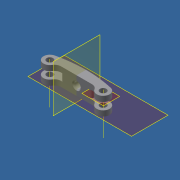
# Autodesk Inventor part: Hebel_B dual
Saved by Autodesk Inventor 2016 (Build 200138000, 138)
## iProperties
Created: 2014-12-22
Part Number: Hebel_B dual
Material: Generisch
Document SubType Name: Modeling
Designer: 4ndreas
Density: 1 g/cm^3
Appearance: Vorgabe
Mass: 1.35892 g
Surface Area: 18.535 cm^2
Volume: 1.35892 cm^3
Author: 4ndreas
Autodesk Inventor part; units mm, degrees
ref_plane "YZ Plane" through (0, 0, 0) normal (1, 0, 0) x (0, 1, 0)
ref_plane "XZ Plane" through (0, 0, 0) normal (0, 1, 0) x (-1, 0, 0)
ref_plane "XY Plane" through (0, 0, 0) normal (0, 0, 1) x (1, 0, 0)
sketch "Skizze1" plane through (0, 0, 0) normal (0, 0, 1) x (1, 0, 0)
  line L0 (0, 0) -> (25, 0) construction
  arc A0 (0, 3) -> (2.5981, -1.5) centre (0, 0) ccw
  arc A1 (22.4019, -1.5) -> (25, 3) centre (25, 0) ccw
  arc A2 (22.4019, -1.5) -> (19.8038, 0) centre (19.8038, -3) ccw
  arc A3 (5.1962, 0) -> (2.5981, -1.5) centre (5.1962, -3) ccw
  line L1 (0, 3) -> (25, 3)
  line L2 (5.1962, 0) -> (19.8038, 0)
  line L3 (12.5, 0) -> (12.5, 11.1623) construction
  line L4 (-0.6713, 2.9239) -> (12.5, 5.9481) construction
  line L5 (12.5, 5.9481) -> (25.6713, 2.9239) construction
  spline S0 degree 2 poles (-0.6713, 2.9239) (12.5, 5.9481) (25.6713, 2.9239) knots 1 1 1 2 2 2
  dimension "d0" = 25
  dimension "d1" = 3
  dimension "d2" = 3
  constraints: 10 point on circle, 8 end point, 8 tangent, 4 centre point, 2 coincident, 1 collinear, 1 equal radius, 1 horizontal, 1 midpoint, 1 parallel, 1 perpendicular, 1 point on line, 4 other
  measures "d0" distance of L0.start L0.end
  measures "d1" radius of A0
  measures "d2" distance between parallel lines of L2 L1
ref_plane "Arbeitsebene1" through (0, 3, 0) normal (0, 0, -1) x (1, 0, 0)
extrude "Extrusion1" add sketch "Skizze1" along normal blind 2.5
sketch "Skizze2" plane through (0, 0, 2.5) normal (0, 0, 1) x (1, 0, 0)
  arc A0 (-0.6713, 2.9239) -> (2.5981, -1.5) centre (0, 0) ccw projected
  arc A1 (22.4019, -1.5) -> (25.6713, 2.9239) centre (25, 0) ccw projected
  point P0 (0, 3)
  point P1 (25, 3)
hole "Bohrung1" at (0, 0, 2.5) at (25, 0, 2.5) direction (0, 0, -1) diameter 3 end through all
sketch "Skizze4" plane through (0, 0, 2.5) normal (0, 0, 1) x (1, 0, 0)
  line L0 (5.1962, 0) -> (19.8038, 0)
  line L1 (5.1962, 0) -> (5.1962, 3.9711)
  line L2 (19.8038, 0) -> (19.8038, 3.9711)
  line L3 (5.1962, 0) -> (19.8038, 0) projected
  spline S0 degree 2 poles (25.6713, 2.9239) (12.5, 5.9481) (-0.6713, 2.9239) knots 0 0 0 1 1 1 projected
  constraints: 6 end point, 1 parallel, 1 perpendicular, 3 other
extrude "Extrusion2" add sketch "Skizze4" along normal blind 1.7
mirror "Spiegeln1" about plane through (12.5, 1.8725, 4.2) normal (0, 0, 1)
fillet "Rundung1" radius 1 2 edges at (5.1962, 0, 4.2) (19.8038, 0, 4.2)
ref_plane "Arbeitsebene2" through (19.8038, 0, 5.65) normal (0, 0, -1) x (-1, 0, 0)
sketch "Skizze5" plane through (19.8038, 0, 5.65) normal (0, 0, -1) x (-1, 0, 0)
  arc A0 (-5.8675, 2.9239) -> (-2.5981, -1.5) centre (-5.1962, 0) ccw construction
  arc A1 (0, 0) -> (-2.5981, -1.5) centre (0, -3) ccw construction
  line L0 (0, 0) -> (1, 0) construction
  arc A2 (0, 1) -> (1, 0) centre (1, 1) ccw construction
  line L1 (0, 3.9711) -> (0, 1) construction
  circle A3 centre (-5.1962, 0) radius 1.5 construction
  line L2 (-8.7757, 6.4711) -> (-0.4769, 6.4711)
  line L3 (-0.4769, 6.4711) -> (-0.4769, -5.5)
  line L4 (-0.4769, -5.5) -> (-8.7757, -5.5)
  line L5 (-8.7757, -5.5) -> (-8.7757, 6.4711)
  line L6 (14.6077, 1) -> (14.6077, 3.9711) projected
  arc A4 (13.6077, 0) -> (14.6077, 1) centre (13.6077, 1) ccw projected
  line L7 (13.6077, 0) -> (14.6077, 0) projected
  arc A5 (17.2058, -1.5) -> (14.6077, 0) centre (14.6077, -3) ccw projected
  arc A6 (17.2058, -1.5) -> (20.4752, 2.9239) centre (19.8038, 0) ccw projected
  dimension "d17" = 2.5
  dimension "d36" = 2.5
  constraints: 8 end point, 2 parallel, 1 horizontal, 1 perpendicular, 2 other
  measures "d17" distance edge to line of A0 L4
  measures "d36" distance from line of L1.start L2
extrude "Extrusion3" add sketch "Skizze5" along normal blind 1.2 separate body
sketch "Skizze6" plane through (19.8038, 0, 4.45) normal (0, 0, -1) x (-1, 0, 0)
  line L0 (-8.7757, -5.5) -> (-0.4769, -5.5) projected
  line L1 (-0.4769, -5.5) -> (-0.4769, 6.4711) projected
  line L2 (-8.7757, 6.4711) -> (-0.4769, 6.4711)
  line L3 (-0.4769, 6.4711) -> (-0.4769, 4.4711)
  line L4 (-0.4769, 4.4711) -> (-8.7757, 4.4711)
  line L5 (-8.7757, 4.4711) -> (-8.7757, 6.4711)
  line L6 (-8.7757, -5.5) -> (-0.4769, -5.5)
  line L7 (-0.4769, -5.5) -> (-0.4769, -3.5)
  line L8 (-0.4769, -3.5) -> (-8.7757, -3.5)
  line L9 (-8.7757, -3.5) -> (-8.7757, -5.5)
  point P0 (19.8038, 0)
  dimension "d20" = 2
  dimension "d21" = 2
  constraints: 16 end point, 4 parallel, 2 horizontal, 2 perpendicular, 2 point on line
  measures "d20" distance between parallel lines of L4 L2
  measures "d21" distance between parallel lines of L0 L8
extrude "Extrusion4" add sketch "Skizze6" along normal up to surface (4.45 mm away)
ref_plane "Arbeitsebene3" through (12.5, 0, 8.4) normal (1, 0, 0) x (0, 1, 0)
mirror "Spiegeln2" about plane through (12.5, 0, 8.4) normal (1, 0, 0) of "Extrusion3", "Extrusion4"
sketch "Skizze7" plane through (5.1962, 0, 0) normal (0, -1, 0) x (1, 0, 0)
  line L0 (1, 2.5) -> (1, 5.9) projected
  line L1 (13.6077, 5.9) -> (13.6077, 2.5) projected
  line L2 (1, 4.2) -> (13.6077, 4.2) construction
  point P0 (-5.1962, 0)
  point P1 (7.3038, 4.2)
  constraints: 3 midpoint, 2 end point
hole "Bohrung2" at (12.5, 0, 4.2) direction (0, 1, 0) diameter 3 end through all countersink diameter 4 countersink angle 90
equation "\"d0\" = Hebel_B"
equation "\"d1\" = FingerWall"
equation "\"d36\" = d17"
equation "\"d21\" = d20"
equation "\"FingerLaenge_B\" = 25"
equation "\"Hebel_B\" = 25"
equation "\"Finger_width\" = 22"
equation "\"Hebel_basis_2\" = 15"
equation "\"Finger_diameter\" = 8"
equation "\"FingerWall\" = 3"
equation "\"Join_width\" = 3"
equation "\"bearingHole\" = 3"
equation "\"bearingWall\" = 4"
equation "\"support_D\" = 0.25"
equation "\"d37\" = support_D"
